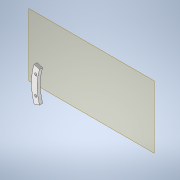
# Autodesk Inventor part: Montage_Ring_Hinten_Aufdickung
Saved by Autodesk Inventor 2022.2 (Build 262287010, 287A)
## iProperties
Created: 2024-01-10
Part Number: Montage_Ring_Hinten_Aufdickung
Material: Generisch
Document SubType Name: Modeling
Designer: ppovolni
Density: 1 g/cm^3
Appearance: Vorgabe
Author: ppovolni
Autodesk Inventor part; units mm, degrees
ref_plane "YZ Plane" through (0, 0, 0) normal (1, 0, 0) x (0, 1, 0)
ref_plane "XZ Plane" through (0, 0, 0) normal (0, 1, 0) x (-1, 0, 0)
ref_plane "XY Plane" through (0, 0, 0) normal (0, 0, 1) x (1, 0, 0)
ref_plane "Arbeitsebene1" through (0, 0, 0) normal (0, 0, 1) x (1, 0, 0)
sketch "Skizze1" plane through (0, 0, 0) normal (0, 0, 1) x (1, 0, 0)
  arc A0 (91.8, -45.9) -> (-91.8, -45.9) centre (0, -45.9) ccw construction
  line L0 (-91.8, -45.9) -> (-80.6, -45.9) construction
  arc A1 (-5.5, 34.5121) -> (-80.6, -45.9) centre (0, -45.9) ccw construction
  line L1 (-5.5, 34.5121) -> (-5.5, 40.0242) construction
  arc A2 (5.5, 40.0242) -> (-5.5, 40.0242) centre (0, -45.9) ccw construction
  line L2 (5.5, 40.0242) -> (5.5, 34.5121) construction
  arc A3 (80.6, -45.9) -> (5.5, 34.5121) centre (0, -45.9) ccw construction
  line L3 (80.6, -45.9) -> (91.8, -45.9) construction
  arc A4 (-91.8, -45.9) -> (91.8, -45.9) centre (0, -45.9) ccw construction
  line L4 (91.8, -45.9) -> (80.6, -45.9) construction
  arc A5 (-80.6, -45.9) -> (80.6, -45.9) centre (0, -45.9) ccw construction
  line L5 (-80.6, -45.9) -> (-91.8, -45.9) construction
  circle A6 centre (-84.8904, -30.9315) radius 2.05
  circle A7 centre (-84.8904, -60.8685) radius 2.05
  circle A8 centre (84.8904, -30.9315) radius 2.05
  circle A9 centre (84.8904, -60.8685) radius 2.05
  arc A10 (-87.5512, -18.2952) -> (-87.5512, -73.5048) centre (0, -45.9) ccw
  line L6 (-87.5512, -18.2952) -> (0, -45.9)
  line L7 (0, -45.9) -> (-87.5512, -73.5048)
  line L8 (-91.8, -45.9) -> (-80.6, -45.9)
  circle A11 centre (84.8904, -60.8685) radius 2.05
  circle A12 centre (-84.8904, -60.8685) radius 2.05
  circle A13 centre (-84.8904, -30.9315) radius 2.05
  circle A14 centre (84.8904, -30.9315) radius 2.05
  arc A15 (-78.777, -21.0617) -> (-78.777, -70.7383) centre (0, -45.9) ccw
  point P0 (0, 0)
  point P1 (-76.8696, -21.6631)
  point P2 (-76.8696, -70.1369)
extrude "Extrusion1" add sketch "Skizze1" along normal blind 5 contours L6 A15 L8 A10 | L8 A15 L7 A10
